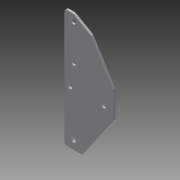
# Autodesk Inventor part: Ninja left cylinder support bracket
Saved by Autodesk Inventor 2014 SP1 (Build 180222100, 222)
## iProperties
Created: 2013-03-16
Part Number: Ninja left cylinder support bracket
Material: Aluminum 6061
Document SubType Name: Modeling
Designer: Arpan
Density: 2.71 g/cm^3
Appearance: Aluminum - Flat
Mass: 74.6186 g
Surface Area: 189.875 cm^2
Volume: 27.5345 cm^3
Author: Arpan
Autodesk Inventor part; units mm, degrees
ref_plane "YZ Plane" through (0, 0, 0) normal (1, 0, 0) x (0, 1, 0)
ref_plane "XZ Plane" through (0, 0, 0) normal (0, 1, 0) x (-1, 0, 0)
ref_plane "XY Plane" through (0, 0, 0) normal (0, 0, 1) x (1, 0, 0)
sketch "Sketch1" plane through (0, 0, 0) normal (0, 0, 1) x (1, 0, 0)
  line L0 (69.85, 0) -> (69.85, 38.1)
  line L1 (69.85, 38.1) -> (29.1042, 104.775)
  line L2 (0, 104.775) -> (0, 0)
  line L3 (0, -63.5) -> (0, 0)
  line L4 (0, 104.775) -> (29.1042, 104.775)
  line L5 (0, -63.5) -> (25.4, -63.5)
  line L6 (25.4, -63.5) -> (69.85, 0)
  dimension "d1" = 38.1
  dimension "d24" = 63.5
  dimension "d25" = 69.85
  dimension "d26" = 69.85
  dimension "d36" = 104.775
  dimension "d38" = 121.43
  dimension "d45" = 25.4
  constraints: 14 end point, 2 parallel, 1 collinear, 1 perpendicular, 1 vertical
  measures "d1" distance of L0.start L0.end
  measures "d24" distance of L3.start L2.end
  measures "d25" distance between parallel lines of L2 L0
  measures "d26" distance of L2.end L0.start
  measures "d36" distance of L2.start L2.end
  measures "d38" angle of L4 L1
  measures "d45" distance of L3.start L5.end
extrude "Extrusion1" add sketch "Sketch1" along normal blind 3.175
sketch "Sketch2" plane through (0, 0, 3.175) normal (0, 0, 1) x (1, 0, 0)
  line L0 (0, 0) -> (69.85, 0) projected
  line L1 (69.85, 0) -> (69.85, 38.1) projected
  line L2 (0, 104.775) -> (0, -63.5) projected
  circle A0 centre (7.874, 12.7) radius 3.556
  circle A1 centre (55.626, 12.7) radius 3.556
  point P0 (0, 152.4)
  dimension "d5" = 7.112
  dimension "d6" = 7.112
  dimension "d7" = 12.7
  dimension "d8" = 12.7
  dimension "d9" = 14.224
  dimension "d11" = 7.874
  constraints: 2 centre point
  measures "d5" diameter of A0
  measures "d6" diameter of A1
  measures "d7" distance from line of L0 A0.centre
  measures "d8" distance from line of L0 A1.centre
  measures "d9" distance from line of L1 A1.centre
  measures "d11" distance from line of A0.centre L2
extrude "Extrusion2" cut sketch "Sketch2" against normal blind 25.4
sketch "Sketch3" plane through (0, 0, 3.175) normal (0, 0, 1) x (1, 0, 0)
  line L0 (0, 104.775) -> (0, -63.5) projected
  line L1 (0, 0) -> (69.85, 0) projected
  circle A0 centre (12.7, 94.9198) radius 3.3782
  circle A1 centre (12.7, 44.1198) radius 3.3782
  point P0 (0, 141.1158)
  dimension "d15" = 6.7564
  dimension "d16" = 6.7564
  dimension "d17" = 12.7
  dimension "d18" = 12.7
  dimension "d19" = 44.1198
  dimension "d20" = 50.8
  constraints: 2 centre point
  measures "d15" diameter of A0
  measures "d16" diameter of A1
  measures "d17" distance from line of L0 A0.centre
  measures "d18" distance from line of L0 A1.centre
  measures "d19" distance from line of A1.centre L1
  measures "d20" distance of A0.centre A1.centre
extrude "Extrusion3" cut sketch "Sketch3" against normal blind 25.4
fillet "Fillet2" radius 3.175 2 edges at (69.85, 0, 1.5875) (69.85, 38.1, 1.5875)
fillet "Fillet3" radius 3.175 1 edges at (0, -63.5, 1.5875)
sketch "Sketch4" plane through (0, 0, 3.175) normal (0, 0, 1) x (1, 0, 0)
  line L0 (0, 104.775) -> (0, -60.325) projected
  circle A0 centre (12.7, 44.1198) radius 3.3782 projected
  circle A1 centre (12.7, -51.1302) radius 3.3782
  point P0 (0, 141.1158)
  point P1 (0, 0)
  dimension "d28" = 6.7564
  dimension "d29" = 95.25
  dimension "d30" = 12.7
  constraints: 1 centre point
  measures "d28" diameter of A1
  measures "d29" distance of A0.centre A1.centre
  measures "d30" distance from line of L0 A1.centre
extrude "Extrusion4" cut sketch "Sketch4" against normal blind 25.4 contours A1
sketch "Sketch5" plane through (0, 0, 3.175) normal (0, 0, 1) x (1, 0, 0)
  circle A0 centre (12.7, 44.1198) radius 3.3782 projected
  circle A1 centre (12.7, 94.9198) radius 3.3782 projected
  point P0 (0, 0)
extrude "Extrusion5" cut sketch "Sketch5" against normal blind 25.4
fillet "Fillet4" radius 3.175 2 edges at (29.1042, 104.775, 1.5875) (0, 104.775, 1.5875)
sketch "Sketch6" plane through (0, 0, 3.175) normal (0, 0, 1) x (1, 0, 0)
  line L0 (0, 101.6) -> (0, -60.325) projected
  line L1 (69.3842, 38.8623) -> (30.0327, 103.2556) projected
  arc A0 (30.0327, 103.2556) -> (27.3235, 104.775) centre (27.3235, 101.6) ccw projected
  line L2 (27.3235, 104.775) -> (3.175, 104.775) projected
  line L3 (12.7, 104.775) -> (38.0473, 90.1407)
  point P0 (0, 0)
  dimension "d40" = 30
  dimension "d41" = 12.7
  constraints: 2 end point, 2 point on line
  measures "d40" angle of L2 L3
  measures "d41" distance from line of L0 L3.start
extrude "Extrusion6" cut sketch "Sketch6" against normal blind 25.4
fillet "Fillet5" radius 3.175 2 edges at (12.7, 104.775, 1.5875) (38.0473, 90.1407, 1.5875)
fillet "Fillet6" radius 3.175 1 edges at (25.4, -63.5, 1.5875)
body "Solid1"
